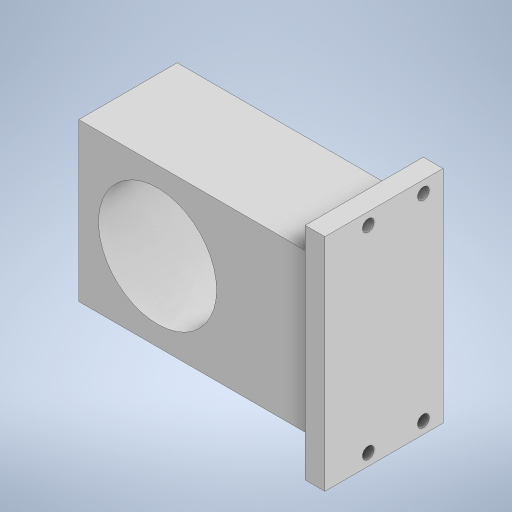
# Autodesk Inventor part: 다리-0
Saved by Autodesk Inventor 2024 (Build 280153000, 153)
## iProperties
Created: 2024-09-10
Part Number: 다리-0
Material: 일반
Document SubType Name: Modeling
Designer: USER
Density: 1 g/cm^3
Appearance: 기본값
Author: USER
Autodesk Inventor part; units mm, degrees
ref_plane "YZ Plane" through (0, 0, 0) normal (1, 0, 0) x (0, 1, 0)
sketch "스케치1" plane through (0, 0, 0) normal (0, 0, 1) x (1, 0, 0)
  line L0 (0, 0) -> (60, 0)
  line L1 (60, 0) -> (60, 40)
  line L2 (60, 40) -> (0, 40)
  line L3 (0, 40) -> (0, 0)
  dimension "d0" = 40
  dimension "d1" = 60
  constraints: 8 end point, 2 parallel, 1 horizontal, 1 perpendicular
  measures "d0" distance of L2.end L0.start
  measures "d1" distance of L1.end L2.end
extrude "돌출1" add sketch "스케치1" along normal blind 25
sketch "스케치2" plane through (0, 0, 25) normal (0, 0, 1) x (1, 0, 0)
  line L0 (60, 0) -> (60, 40) projected
  line L1 (60, 40) -> (0, 40) projected
  line L2 (0, 40) -> (0, 0) projected
  line L3 (0, 0) -> (60, 0) projected
  circle A0 centre (20, 20) radius 15
  point P0 (0, 20)
  dimension "d4" = 30
  dimension "d5" = 20
  constraints: 1 centre point, 1 horizontal alignment, 1 midpoint
  measures "d4" diameter of A0
  measures "d5" distance from line of L2 A0.centre
extrude "돌출2" cut sketch "스케치2" against normal through all contours A0
ref_plane "작업 평면1" through (0, 0, 12.5) normal (0, 0, 1) x (1, 0, 0)
ref_plane "작업 평면2" through (0, 20, 0) normal (0, -1, 0) x (1, 0, 0)
sketch "스케치3" plane through (60, 0, 0) normal (1, 0, 0) x (0, 0, -1)
  line L0 (0, 0) -> (0, 40) projected
  line L1 (0, 40) -> (-25, 40) projected
  line L2 (-25, 0) -> (-25, 40) projected
  line L3 (0, 0) -> (-25, 0) projected
  line L4 (-27.5, 0) -> (2.5, 0)
  line L5 (2.5, 0) -> (2.5, 40)
  line L6 (2.5, 40) -> (-27.5, 40)
  line L7 (-27.5, 40) -> (-27.5, 0)
  line L8 (-27.5, -8) -> (2.5, -8)
  line L9 (2.5, -8) -> (2.5, 48)
  line L10 (2.5, 48) -> (-27.5, 48)
  line L11 (-27.5, 48) -> (-27.5, -8)
  circle A0 centre (-16.5, -5) radius 1.5
  circle A1 centre (-2.5, -5) radius 1.5
  circle A2 centre (-16.5, 45) radius 1.5
  circle A3 centre (-2.5, 45) radius 1.5
  point P0 (0, 0)
  point P1 (-12.5, 0)
  point P2 (-12.5, 0)
  point P3 (-27.5, 20)
  point P4 (-25, 20)
  point P5 (-27.5, 0)
  point P6 (2.5, 0)
  dimension "d8" = 40
  dimension "d9" = 30
  dimension "d10" = 8
  dimension "d11" = 8
  dimension "d12" = 30
  dimension "d13" = 3
  dimension "d14" = 3
  dimension "d15" = 3
  dimension "d16" = 3
  dimension "d17" = 5
  dimension "d18" = 5
  dimension "d19" = 14
  dimension "d20" = 5
  constraints: 16 end point, 4 centre point, 4 midpoint, 4 parallel, 3 horizontal alignment, 2 horizontal, 2 perpendicular, 2 vertical alignment, 1 coincident, 1 point on line
  measures "d8" distance of L6.end L4.start
  measures "d9" distance between parallel lines of L5 L7
  measures "d10" distance between parallel lines of L3 L8
  measures "d11" distance between parallel lines of L10 L1
  measures "d12" distance between parallel lines of L7 L9
  measures "d13" diameter of A0
  measures "d14" diameter of A1
  measures "d15" diameter of A2
  measures "d16" diameter of A3
  measures "d17" distance from line of L3 A0.centre
  measures "d18" distance from line of L6 A2.centre
  measures "d19" distance of A1.centre A0.centre
  measures "d20" distance from line of L5 A1.centre
extrude "돌출3" add sketch "스케치3" along normal blind 5
